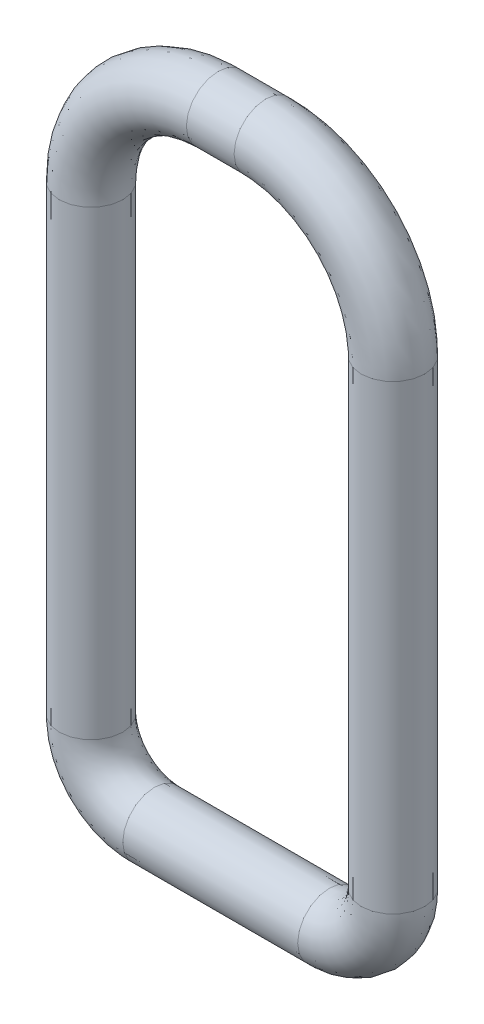
# Autodesk Inventor part: Schlauchoot
Saved by Autodesk Inventor 2020.3 (Build 243373000, 373)
## iProperties
Created: 2020-02-10
Part Number: Schlauchoot
Material: Generisch
Document SubType Name: Modeling
Designer: Stefan
Density: 1 g/cm^3
Appearance: Vorgabe
Author: Stefan
Autodesk Inventor part; units mm, degrees
ref_plane "YZ Plane" through (0, 0, 0) normal (1, 0, 0) x (0, 1, 0)
ref_plane "XZ Plane" through (0, 0, 0) normal (0, 1, 0) x (-1, 0, 0)
ref_plane "XY Plane" through (0, 0, 0) normal (0, 0, 1) x (1, 0, 0)
sketch "Skizze2" plane through (0, 0, 0) normal (0, 0, 1) x (1, 0, 0)
  line L0 (2025.4005, -231.4718) -> (2025.4005, 1218.5282)
  line L1 (1625.4005, 1618.5282) -> (1475.4005, 1618.5282)
  line L2 (1075.4005, 1218.5282) -> (1075.4005, -231.4718)
  arc A0 (1077.4005, 1618.5282) -> (1075.4005, 1616.5282) centre (1077.4005, 1616.5282) ccw
  arc A1 (1475.4005, 1618.5282) -> (1075.4005, 1218.5282) centre (1475.4005, 1218.5282) ccw
  arc A2 (2025.4005, 1218.5282) -> (1625.4005, 1618.5282) centre (1625.4005, 1218.5282) ccw
  arc A3 (1075.4005, -231.4718) -> (1275.4005, -431.4718) centre (1275.4005, -231.4718) ccw
  arc A4 (1825.4005, -431.4718) -> (2025.4005, -231.4718) centre (1825.4005, -231.4718) ccw
  line L3 (1825.4005, -431.4718) -> (1275.4005, -431.4718)
  point P0 (0, 0)
  point P1 (2025.4005, 1618.5282)
  point P2 (2025.4005, -331.4718)
  point P3 (1075.4005, 1618.5282)
  dimension "d2" = 950
  dimension "d3" = 1950
  dimension "d4" = 2
  dimension "d5" = 400
  dimension "d6" = 200
  dimension "d16" = 1450
  dimension "d17" = 1450
  constraints: 11 point on circle, 8 end point, 8 tangent, 7 point on line, 5 centre point, 2 equal radius, 1 horizontal, 1 parallel
  measures "d2" distance of point (1075.401, 1618.528) point (2025.401, 1618.528)
  measures "d3" distance of point (2025.401, 1618.528) point (2025.401, -331.472)
  measures "d4" radius of A0
  measures "d5" radius of A1
  measures "d6" radius of A3
  measures "d16" distance of L0.start L0.end
  measures "d17" distance of L2.start L2.end
sketch "Skizze4" plane through (0, 0, 0) normal (0, 1, 0) x (-1, 0, 0)
  circle A0 centre (-1075.6958, 0) radius 100
  point P0 (0, 0)
  dimension "d11" = 200
  constraints: 1 centre point
  measures "d11" diameter of A0
sweep "Sweeping1" add profiles "Skizze4" path "Skizze2" path curves L3 A4 L0 A2 L1 A1 L2 A3
